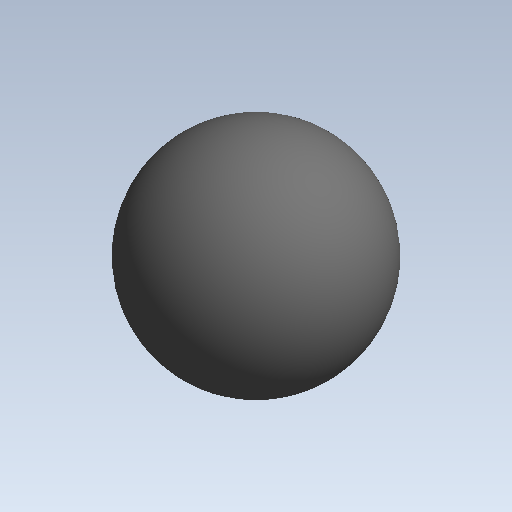
# Autodesk Inventor part: MR106ZZ1 Ball
Saved by Autodesk Inventor 2021.3 (Build 253353010, 353A)
## iProperties
Part Number: MR106ZZ1 Ball
Material: 一般
Catalog Web Link: www.cadenas.de
Description: shielde_type_zz_zzs_B-
Vendor: NSK_RB
Document SubType Name: Modeling
Designer: partserver
Manufacturer: NSK_RB
Mass: 0.000904779 g
Surface Area: 0.0452389 cm^2
Volume: 0.000904779 cm^3
Density: 1 g/cm^3
Appearance: PSOLRGB-128-128-128
Category: PARTsolutions
Company: NSK_RB
PSOL_IDENT_0: {$CADENAS_DATA\23d-libs\nsk_rb\roller_bearings\deep_groove_bb\exstra_small_miniatur_bb\metric_design
PSOL_IDENT_1: \shielded_type_zz_zzs_b.prj},182 {VTYP=3D},{NB=MR106ZZ1 Ball},{LINA=MR106ZZ1 Ball},{NN=shielde_type_
PSOL_IDENT_2: zz_zzs_B},{DATE=25.05.2021 06:41:25},{GEOMDATE=04.01.2008 00:00:00},{VERSION=},{LINEID=600},{WBVAR=}
PSOL_IDENT_3: ,{WBNUMERIC=}  {NB=MR106ZZ1 Ball},{LINA=MR106ZZ1 Ball},{KT=DUMMY},{IDNR=},{STAN=Standard},{ORDER=MR1
PSOL_IDENT_4: 06ZZ1},{SD=6.0},{X=6.0},{DI1=7.04},{DI2=7.04},{SDE1=8.90},{SDE2=9.25},{D=10},{DD=10},{B=0.0},{B1=3.0
PSOL_IDENT_5: },{R=0.00},{R1=0.10},{CR1=495},{COR1=218},{CR2=51},{COR2=22.0},{LG=45000},{LO=53000},{DA=0.0},{DB=7.
PSOL_IDENT_6: 0},{DA1=0.0},{DB1=9.3},{RA=0.00},{RB=0.10},{MASS=0.68},{SC=1}
NB: MR106ZZ1 Ball
NN: shielde_type_zz_zzs_B
NBSYN: $ORDER. Ball
LINA: MR106ZZ1 Ball
CATALOG: NSK Rolling Bearing
STAN: Standard
ORDER: MR106ZZ1
SD: 6
X: 6
DI1: 7.04
DI2: 7.04
SDE1: 8.9
SDE2: 9.25
D: 10
DD: 10
B: 0
B1: 3
R: 0
R1: 0.1
CR1: 495
COR1: 218
CR2: 51
COR2: 22
LG: 45000
LO: 53000
DA: 0
DB: 7
DA1: 0
DB1: 9.3
RA: 0
RB: 0.1
MASS: 0.68
SC: 1
SUPPLIER: NSK_RB
ARTICLENO: MR106ZZ1 Ball
BOMINFO: MR106ZZ1 Ball
CREATOR: CADENAS GmbH
Title: MR106ZZ1 Ball
Author: Cadenas PARTsolutions
Autodesk Inventor part; units mm, degrees
sketch "Sketch_1" plane through (0, 0, 0) normal (0, 0, 1) x (1, 0, 0)
  line L0 (0.6, 0) -> (-0.6, 0)
  arc A0 (0.6, 0) -> (-0.6, 0) centre (0, 0) ccw
  line L1 (0.6, 0) -> (-0.6, 0)
  constraints: 4 end point, 2 point on circle, 1 centre point
revolve "Revolution1" add sketch "Sketch_1" angle 360 about axis through (0.6, 0, 0) along (1, 0, 0)
ref_plane "ip_st_b_XY" through (0, 0, 0) normal (-1, 0, 0) x (0, 0, -1)
ref_plane "ip_st_b_YZ" through (0, 0, 0) normal (0, 0, -1) x (0, -1, 0)
ref_plane "ip_st_b_ZX" through (0, 0, 0) normal (0, -1, 0) x (-1, 0, 0)
body "Solid1"
